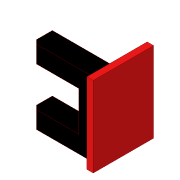
# Autodesk Inventor part: SYS IR Sensor
Saved by Autodesk Inventor 2017 (Build 210142000, 142)
## iProperties
Part Number: SYS IR Sensor
Material: Generisch
Document SubType Name: Modeling
Designer: Werkstatt
Density: 1 g/cm^3
Appearance: Vorgabe(1)
Author: Werkstatt
Autodesk Inventor part; units mm, degrees
ref_plane "YZ Plane" through (0, 0, 0) normal (1, 0, 0) x (0, 1, 0)
ref_plane "XZ Plane" through (0, 0, 0) normal (0, 1, 0) x (-1, 0, 0)
ref_plane "XY Plane" through (0, 0, 0) normal (0, 0, 1) x (1, 0, 0)
sketch "Skizze1" plane through (0, 0, 0) normal (0, 1, 0) x (-1, 0, 0)
  line L0 (0, 0) -> (13.65, 0) construction
  line L1 (15.3, 9.35) -> (0, 9.35)
  line L2 (3.6, 5) -> (15.3, 5)
  line L3 (15.3, 5) -> (15.3, 9.35)
  line L4 (0, 9.35) -> (3.95, 9.35)
  line L5 (3.6, 5) -> (3.6, -5)
  line L6 (3.95, -9.35) -> (0, -9.35)
  line L7 (0, -9.35) -> (0, 9.35)
  line L8 (0, -9.35) -> (15.3, -9.35)
  line L9 (15.3, -9.35) -> (15.3, -5)
  line L10 (15.3, -5) -> (3.6, -5)
  dimension "d0" = 18.7
  dimension "d1" = 10
  dimension "d2" = 15.3
  dimension "d3" = 3.6
  constraints: 22 end point, 4 horizontal, 4 parallel, 2 perpendicular, 1 collinear, 1 midpoint, 1 point on line, 2 other
  measures "d0" diameter of L1 L0
  measures "d1" diameter of L2 L0
  measures "d2" distance between parallel lines of L7 L9
  measures "d3" distance between parallel lines of L7 L5
extrude "Extrusion1" add sketch "Skizze1" along normal blind 5
sketch "Skizze3" plane through (0, 0, 0) normal (1, 0, 0) x (0, 1, 0)
  line L0 (0, 9.35) -> (0, -9.35) projected
  line L1 (0, -9.35) -> (5, -9.35) projected
  line L2 (5, 9.35) -> (5, -9.35) projected
  line L3 (0, 9.35) -> (5, 9.35) projected
  line L4 (13.7, 10.15) -> (-1.55, 10.15)
  line L5 (-1.55, 10.15) -> (-1.55, -10.15)
  line L6 (-1.55, -10.15) -> (13.7, -10.15)
  line L7 (13.7, -10.15) -> (13.7, 10.15)
  line L8 (0, 0) -> (5, 0) construction
  dimension "d6" = 15.25
  dimension "d7" = 20.3
  dimension "d8" = 8.7
  dimension "d9" = 1.55
  constraints: 10 end point, 2 parallel, 1 horizontal, 1 midpoint, 1 perpendicular, 1 other
  measures "d6" distance of L5.end L6.end
  measures "d7" distance of L6.end L4.start
  measures "d8" distance between parallel lines of L2 L7
  measures "d9" distance between parallel lines of L5 L0
extrude "Extrusion2" add sketch "Skizze3" along normal blind 1.6 contours L3 L2 L1 L0 | L7 L6 L5 L4
chamfer "Fase1" distance 1 angle 45 2 edges at (-15.3, 0, -7.175) (-15.3, 0, 7.175)
